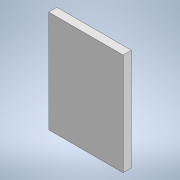
# Autodesk Inventor part: bussola
Saved by Autodesk Inventor 2022.1 (Build 261234000, 234)
## iProperties
Created: 2021-07-07
Part Number: bussola
Material: Generic
Document SubType Name: Modeling
Designer: dwbertol
Density: 1 g/cm^3
Appearance: Default
Author: dwbertol
Autodesk Inventor part; units mm, degrees
ref_plane "YZ Plane" through (0, 0, 0) normal (1, 0, 0) x (0, 1, 0)
ref_plane "XZ Plane" through (0, 0, 0) normal (0, 1, 0) x (-1, 0, 0)
ref_plane "XY Plane" through (0, 0, 0) normal (0, 0, 1) x (1, 0, 0)
sketch "Sketch1" plane through (0, 0, 0) normal (0, 0, 1) x (1, 0, 0)
  line L0 (-5.7378, 10.9988) -> (7.7622, 10.9988)
  line L1 (7.7622, 10.9988) -> (7.7622, -7.5012)
  line L2 (7.7622, -7.5012) -> (-5.7378, -7.5012)
  line L3 (-5.7378, -7.5012) -> (-5.7378, 10.9988)
  point P0 (0, 0)
  dimension "d0" = 13.5
  dimension "d1" = 18.5
  constraints: 8 end point, 2 parallel, 1 horizontal, 1 perpendicular
  measures "d0" distance of L1.end L2.end
  measures "d1" distance of L0.end L1.end
extrude "Extrusion1" add sketch "Sketch1" along normal blind 1.5
body "Solid1"
